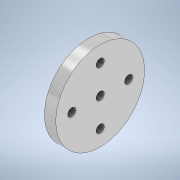
# Autodesk Inventor part: Part R
Saved by Autodesk Inventor 2021 (Build 250183000, 183)
## iProperties
Created: 2021-10-22
Part Number: Part R
Material: Generic
Document SubType Name: Modeling
Designer: Asus
Density: 1 g/cm^3
Appearance: Default
Author: Asus
Autodesk Inventor part; units mm, degrees
ref_plane "YZ Plane" through (0, 0, 0) normal (1, 0, 0) x (0, 1, 0)
ref_plane "XZ Plane" through (0, 0, 0) normal (0, 1, 0) x (-1, 0, 0)
ref_plane "XY Plane" through (0, 0, 0) normal (0, 0, 1) x (1, 0, 0)
sketch "Sketch1" plane through (0, 0, 0) normal (1, 0, 0) x (0, 1, 0)
  circle A0 centre (0, 0) radius 10.9
  circle A1 centre (0, 0) radius 1
  circle A2 centre (0, 0) radius 7
  circle A3 centre (7, 0) radius 1
  circle A4 centre (0, 7) radius 1
  circle A5 centre (-7, 0) radius 1
  circle A6 centre (0, -7) radius 1
  dimension "d2" = 14
  dimension "d0" = 21.8
  dimension "d1" = 2
  dimension "d3" = 2
  dimension "d6" = 360
  constraints: 6 centre point, 3 coincident, 1 horizontal alignment, 11 other
  measures "d0" diameter of A0
  measures "d1" diameter of A1
  measures "d3" diameter of A3
extrude "Extrusion1" add sketch "Sketch1" along normal blind 2.8 contours A0 | A3 A2 A6 A5 A4
sketch "Sketch2" plane through (0, 0, 0) normal (-1, 0, 0) x (0, 0, 1)
  circle A0 centre (0, 0) radius 3.5
  line L0 (-0.0024, 0.0008) -> (1.8342, 0.0008) construction
  line L1 (0, 0) -> (2, 0) construction
  circle A1 centre (0, 0) radius 1.8335
  line L2 (-0.517, -1.932) -> (-0.6271, -1.7229)
  line L3 (-0.517, -1.932) -> (-0.3208, -1.8052)
  line L4 (-0.1736, -1.9924) -> (-0.3184, -1.8056)
  line L5 (-0.1736, -1.9924) -> (-0.0025, -1.8335)
  line L6 (0.175, -1.9923) -> (0, -1.8335)
  line L7 (0.175, -1.9923) -> (0.316, -1.806)
  line L8 (0.5183, -1.9317) -> (0.3184, -1.8056)
  line L9 (0.5183, -1.9317) -> (0.6248, -1.7237)
  line L10 (0.8458, -1.8123) -> (0.6271, -1.7229)
  line L11 (0.8458, -1.8123) -> (0.9146, -1.5891)
  line L12 (1.1477, -1.6379) -> (0.9167, -1.5878)
  line L13 (1.1477, -1.6379) -> (1.1766, -1.4061)
  line L14 (1.4147, -1.4137) -> (1.1785, -1.4045)
  line L15 (1.4147, -1.4137) -> (1.4029, -1.1804)
  line L16 (1.6387, -1.1466) -> (1.4045, -1.1785)
  line L17 (1.6387, -1.1466) -> (1.5866, -0.9189)
  line L18 (1.8129, -0.8446) -> (1.5878, -0.9167)
  line L19 (1.8129, -0.8446) -> (1.7221, -0.6294)
  line L20 (1.932, -0.517) -> (1.7229, -0.6271)
  line L21 (1.932, -0.517) -> (1.8052, -0.3208)
  line L22 (1.9924, -0.1736) -> (1.8056, -0.3184)
  line L23 (1.9924, -0.1736) -> (1.8335, -0.0025)
  line L24 (1.9923, 0.175) -> (1.8335, 0)
  line L25 (1.9923, 0.175) -> (1.806, 0.316)
  line L26 (1.9317, 0.5183) -> (1.8056, 0.3184)
  line L27 (1.9317, 0.5183) -> (1.7237, 0.6248)
  line L28 (1.8123, 0.8458) -> (1.7229, 0.6271)
  line L29 (1.8123, 0.8458) -> (1.5891, 0.9146)
  line L30 (1.6379, 1.1477) -> (1.5878, 0.9167)
  line L31 (1.6379, 1.1477) -> (1.4061, 1.1766)
  line L32 (1.4137, 1.4147) -> (1.4045, 1.1785)
  line L33 (1.4137, 1.4147) -> (1.1804, 1.4029)
  line L34 (1.1466, 1.6387) -> (1.1785, 1.4045)
  line L35 (1.1466, 1.6387) -> (0.9189, 1.5866)
  line L36 (0.8446, 1.8129) -> (0.9167, 1.5878)
  line L37 (0.8446, 1.8129) -> (0.6294, 1.7221)
  line L38 (0.517, 1.932) -> (0.6271, 1.7229)
  line L39 (0.517, 1.932) -> (0.3208, 1.8052)
  line L40 (0.1736, 1.9924) -> (0.3184, 1.8056)
  line L41 (0.1736, 1.9924) -> (0.0025, 1.8335)
  line L42 (-0.175, 1.9923) -> (0, 1.8335)
  line L43 (-0.175, 1.9923) -> (-0.316, 1.806)
  line L44 (-0.5183, 1.9317) -> (-0.3184, 1.8056)
  line L45 (-0.5183, 1.9317) -> (-0.6248, 1.7237)
  line L46 (-0.8458, 1.8123) -> (-0.6271, 1.7229)
  line L47 (-0.8458, 1.8123) -> (-0.9146, 1.5891)
  line L48 (-1.1477, 1.6379) -> (-0.9167, 1.5878)
  line L49 (-1.1477, 1.6379) -> (-1.1766, 1.4061)
  line L50 (-1.4147, 1.4137) -> (-1.1785, 1.4045)
  line L51 (-1.4147, 1.4137) -> (-1.4029, 1.1804)
  line L52 (-1.6387, 1.1466) -> (-1.4045, 1.1785)
  line L53 (-1.6387, 1.1466) -> (-1.5866, 0.9189)
  line L54 (-1.8129, 0.8446) -> (-1.5878, 0.9167)
  line L55 (-1.8129, 0.8446) -> (-1.7221, 0.6294)
  line L56 (-1.932, 0.517) -> (-1.7229, 0.6271)
  line L57 (-1.932, 0.517) -> (-1.8052, 0.3208)
  line L58 (-1.9924, 0.1736) -> (-1.8056, 0.3184)
  line L59 (-1.9924, 0.1736) -> (-1.8335, 0.0025)
  line L60 (-1.9923, -0.175) -> (-1.8335, 0)
  line L61 (-1.9923, -0.175) -> (-1.806, -0.316)
  line L62 (-1.9317, -0.5183) -> (-1.8056, -0.3184)
  line L63 (-1.9317, -0.5183) -> (-1.7237, -0.6248)
  line L64 (-1.8123, -0.8458) -> (-1.7229, -0.6271)
  line L65 (-1.8123, -0.8458) -> (-1.5891, -0.9146)
  line L66 (-1.6379, -1.1477) -> (-1.5878, -0.9167)
  line L67 (-1.6379, -1.1477) -> (-1.4061, -1.1766)
  line L68 (-1.4137, -1.4147) -> (-1.4045, -1.1785)
  line L69 (-1.4137, -1.4147) -> (-1.1804, -1.4029)
  line L70 (-1.1466, -1.6387) -> (-1.1785, -1.4045)
  line L71 (-1.1466, -1.6387) -> (-0.9189, -1.5866)
  line L72 (-0.8446, -1.8129) -> (-0.9167, -1.5878)
  line L73 (-0.8446, -1.8129) -> (-0.6294, -1.7221)
  arc A2 (2, 0) -> (1.9998, 0.0261) centre (0, 0) ccw
  point P0 (1.8335, 0)
  dimension "d10" = 7
  dimension "d13" = 360
  constraints: 148 end point, 2 centre point, 2 coincident, 2 horizontal, 2 point on circle, 2 point on line, 185 other
  measures "d10" diameter of A0
extrude "Extrusion2" add sketch "Sketch2" along normal blind 2.2
thread "Thread1" size "M2x0.4" class "6H" standard "ANSI Metric M Profile" length 5
thread "Thread2" size "M2x0.4" class "6H" standard "ANSI Metric M Profile" length 5
thread "Thread3" size "M2x0.4" class "6H" standard "ANSI Metric M Profile" length 5
thread "Thread4" size "M2x0.4" class "6H" standard "ANSI Metric M Profile" length 5
thread "Thread5" size "M2x0.4" class "6H" standard "ANSI Metric M Profile" length 5
body "Solid1"
